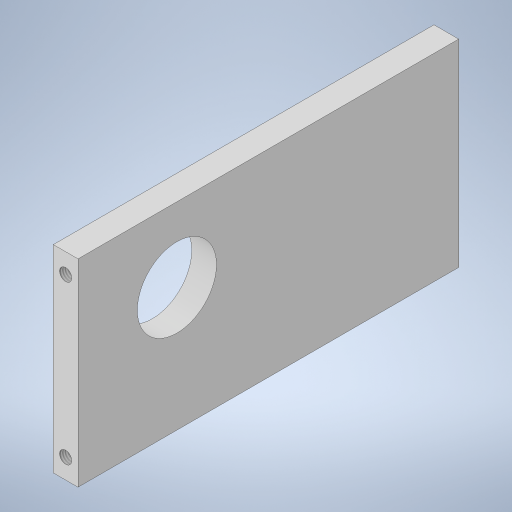
# Autodesk Inventor part: shoulder1_verticval_cover
Saved by Autodesk Inventor 2024 (Build 280153000, 153)
## iProperties
Created: 2025-08-06
Part Number: shoulder1_verticval_cover
Material: 一般
Document SubType Name: Modeling
Designer: HosodaLab2
Density: 1 g/cm^3
Appearance: 既定
Author: HosodaLab2
Autodesk Inventor part; units mm, degrees
ref_plane "YZ Plane" through (0, 0, 0) normal (1, 0, 0) x (0, 1, 0)
ref_plane "XZ Plane" through (0, 0, 0) normal (0, 1, 0) x (-1, 0, 0)
ref_plane "XY Plane" through (0, 0, 0) normal (0, 0, 1) x (1, 0, 0)
sketch "スケッチ2" plane through (0, 0, 0) normal (0, 1, 0) x (-1, 0, 0)
  line L0 (0, 0) -> (-77, 0)
  line L1 (-77, 0) -> (-77, -40)
  line L2 (-77, -40) -> (0, -40)
  line L3 (0, -40) -> (0, 0)
  dimension "d0" = 77
  dimension "d1" = 40
  constraints: 8 end point, 2 parallel, 1 horizontal, 1 perpendicular
  measures "d0" distance of L2.end L1.end
  measures "d1" distance of L1.end L0.end
extrude "押し出し1" add sketch "スケッチ2" along normal blind 5
sketch "スケッチ4" plane through (0, 0, -40) normal (-1, 0, 0) x (0, 0, 1)
  line L0 (0, 0) -> (0, 5) construction
  line L1 (0, 2.5) -> (40, 2.5) construction
  line L2 (40, 0) -> (40, 5) construction
  point P0 (4, 2.5)
  point P1 (36, 2.5)
  dimension "d4" = 4
  dimension "d5" = 4
  constraints: 2 end point, 2 midpoint, 2 point on line
  measures "d4" distance from line of L2 point (36, 2.5)
  measures "d5" distance from line of point (4, 2.5) L0
hole "穴1" at (0, 2.5, -36) at (0, 2.5, -4) direction (1, 0, 0) diameter 2.459 depth 20 thread size "M3x0.5" class "6H" standard "ISO Metric profile"
sketch "スケッチ5" plane through (77, 0, 0) normal (1, 0, 0) x (0, 0, -1)
  line L0 (0, 0) -> (0, 5) construction
  line L1 (0, 2.5) -> (39.9198, 2.5) construction
  circle A0 centre (4, 2.5) radius 1.2295 construction
  circle A1 centre (36, 2.5) radius 1.2295 projected
  constraints: 2 coincident, 2 end point, 1 horizontal, 1 midpoint
hole "穴2" at (77, 2.5, -4) at (77, 2.5, -36) direction (-1, 0, 0) diameter 2.459 depth 20 thread size "M3x0.5" class "6H" standard "ISO Metric profile"
sketch "スケッチ6" plane through (0, 5, 0) normal (0, 1, 0) x (1, 0, 0)
  line L0 (77, 0) -> (77, 40) construction
  line L1 (0, 40) -> (0, 0) construction
  line L2 (0, 0) -> (77, 0) construction
  point P0 (57, 15)
  dimension "d20" = 20
  dimension "d21" = 15
  measures "d20" distance from line of L0 point (57, 15)
  measures "d21" distance from line of L2 point (57, 15)
hole "穴3" at (57, 5, -15) direction (0, -1, 0) diameter 16 end through all
